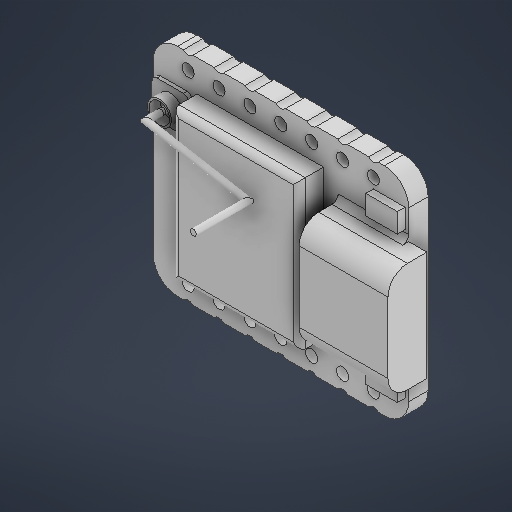
# Autodesk Inventor part: ESP32-S3
Saved by Autodesk Inventor 2027 (Build 310192000, 192)
## iProperties
Created: 2026-07-03
Part Number: ESP32-S3
Material: Genérico
Document SubType Name: Modeling
Designer: marcu
Density: 1 g/cm^3
Appearance: Padrão
Mass: 1.03876 g
Surface Area: 11.537 cm^2
Volume: 1.03876 cm^3
Author: marcu
Autodesk Inventor part; units mm, degrees
ref_plane "YZ Plane" through (0, 0, 0) normal (1, 0, 0) x (0, 1, 0)
ref_plane "XZ Plane" through (0, 0, 0) normal (0, 1, 0) x (-1, 0, 0)
sketch "Esboço1" plane through (0, 0, 0) normal (0, 0, 1) x (1, 0, 0)
  line L0 (-10.5, 8.9) -> (10.5, 8.9)
  line L1 (10.5, 8.9) -> (10.5, -8.9)
  line L2 (10.5, -8.9) -> (-10.5, -8.9)
  line L3 (-10.5, -8.9) -> (-10.5, 8.9)
  line L4 (-10.5, 8.9) -> (10.5, -8.9) construction
  line L5 (10.5, 8.9) -> (-10.5, -8.9) construction
  point P0 (0, 0)
  dimension "d0" = 21
  dimension "d1" = 17.8
  constraints: 12 end point, 2 midpoint, 2 parallel, 1 horizontal, 1 perpendicular
  measures "d0" distance of L1.end L2.end
  measures "d1" distance of L0.end L1.end
extrude "Extrusão1" add sketch "Esboço1" along normal mid plane 1.6
sketch "Esboço2" plane through (0, 0, 0.8) normal (0, 0, 1) x (1, 0, 0)
  line L0 (-23.9402, 0) -> (23.9402, 0) construction
  circle A0 centre (-7.63, 7.62) radius 0.5
  line L1 (-10.5, 8.9) -> (-10.5, -8.9) projected
  line L2 (10.5, 8.9) -> (-10.5, 8.9) projected
  circle A1 centre (-5.09, 7.62) radius 0.5
  circle A2 centre (-2.55, 7.62) radius 0.5
  circle A3 centre (-0.01, 7.62) radius 0.5
  circle A4 centre (2.53, 7.62) radius 0.5
  circle A5 centre (5.07, 7.62) radius 0.5
  circle A6 centre (7.61, 7.62) radius 0.5
  circle A7 centre (-7.63, -7.62) radius 0.5
  line L3 (10.5, -8.9) -> (-10.5, -8.9)
  circle A8 centre (-5.09, -7.62) radius 0.5
  circle A9 centre (-2.55, -7.62) radius 0.5
  circle A10 centre (-0.01, -7.62) radius 0.5
  circle A11 centre (2.53, -7.62) radius 0.5
  circle A12 centre (5.07, -7.62) radius 0.5
  circle A13 centre (7.61, -7.62) radius 0.5
  point P0 (0, 0)
  dimension "d4" = 1
  dimension "d13" = 2.87
  dimension "d14" = 1.28
  dimension "d17" = 2.54
  constraints: 14 centre point, 8 symmetric about line, 4 end point, 2 horizontal, 1 midpoint, 19 other
  measures "d4" diameter of A0
  measures "d13" distance from line of L1 A0.centre
  measures "d14" distance from line of L2 A0.centre
  measures "d17" distance of A0.centre A1.centre
extrude "Extrusão2" cut sketch "Esboço2" against normal blind 2
fillet "Arredondamento1" radius 2 2 edges at (-10.5, 8.9, 0) (-10.5, -8.9, 0)
fillet "Arredondamento2" radius 2 2 edges at (10.5, -8.9, 0) (10.5, 8.9, 0)
sketch "Esboço3" plane through (0, 0, 0.8) normal (0, 0, 1) x (1, 0, 0)
  line L0 (12, -11.9784) -> (12, 11.9784) construction
  line L1 (10.5, -6.9) -> (10.5, 6.9) projected
  line L2 (12, -4.5) -> (4.7, -4.5)
  line L3 (4.7, -4.5) -> (4.7, 4.5)
  line L4 (4.7, 4.5) -> (12, 4.5)
  line L5 (12, 4.5) -> (12, -4.5)
  line L6 (-8.5, -8.9) -> (8.5, -8.9) projected
  point P0 (0, 0)
  dimension "d26" = 1.5
  dimension "d27" = 9
  dimension "d28" = 7.3
  dimension "d29" = 4.4
  constraints: 10 end point, 2 parallel, 2 perpendicular, 1 point on line, 1 vertical
  measures "d26" distance between parallel lines of L1 L0
  measures "d27" distance of L2.end L3.end
  measures "d28" distance of L2.start L2.end
  measures "d29" distance between parallel lines of L2 L6
extrude "Extrusão3" add sketch "Esboço3" along normal blind 3.2
fillet "Arredondamento4" radius 1.6 2 edges at (8.35, 4.5, 4) (8.35, -4.5, 4)
fillet "Arredondamento5" radius 0.5 2 edges at (7.6, -4.5, 0.8) (7.6, 4.5, 0.8)
sketch "Esboço4" plane through (0, 0, 0.8) normal (0, 0, 1) x (1, 0, 0)
  line L0 (-8.5, -8.9) -> (8.5, -8.9) projected
  circle A0 centre (7.61, -9.22) radius 0.5
  line L1 (8.3896, -8.72) -> (6.8304, -8.72) construction
  circle A1 centre (7.61, -7.62) radius 0.5 projected
  line L2 (8.5997, -8.12) -> (6.6203, -8.12) construction
  line L3 (10.5, -6.9) -> (10.5, -5) projected
  circle A2 centre (5.07, -9.22) radius 0.5
  line L4 (5.8496, -8.72) -> (4.2904, -8.72) construction
  circle A3 centre (2.53, -9.22) radius 0.5
  line L5 (3.3096, -8.72) -> (1.7504, -8.72) construction
  circle A4 centre (-0.01, -9.22) radius 0.5
  line L6 (0.7696, -8.72) -> (-0.7896, -8.72) construction
  circle A5 centre (-2.55, -9.22) radius 0.5
  line L7 (-1.7704, -8.72) -> (-3.3296, -8.72) construction
  circle A6 centre (-5.09, -9.22) radius 0.5
  line L8 (-4.3104, -8.72) -> (-5.8696, -8.72) construction
  circle A7 centre (-7.63, -9.22) radius 0.5
  line L9 (-6.8504, -8.72) -> (-8.4096, -8.72) construction
  line L10 (2.05, 0) -> (-2.05, 0) construction
  line L11 (-8.5, 8.9) -> (8.5, 8.9)
  circle A8 centre (7.61, 9.22) radius 0.5
  line L12 (8.3896, 8.72) -> (6.8304, 8.72) construction
  circle A9 centre (5.07, 9.22) radius 0.5
  line L13 (5.8496, 8.72) -> (4.2904, 8.72) construction
  circle A10 centre (2.53, 9.22) radius 0.5
  line L14 (3.3096, 8.72) -> (1.7504, 8.72) construction
  circle A11 centre (-0.01, 9.22) radius 0.5
  line L15 (0.7696, 8.72) -> (-0.7896, 8.72) construction
  circle A12 centre (-2.55, 9.22) radius 0.5
  line L16 (-1.7704, 8.72) -> (-3.3296, 8.72) construction
  circle A13 centre (-5.09, 9.22) radius 0.5
  line L17 (-4.3104, 8.72) -> (-5.8696, 8.72) construction
  circle A14 centre (-7.63, 9.22) radius 0.5
  line L18 (-6.8504, 8.72) -> (-8.4096, 8.72) construction
  point P0 (0, 0)
  point P1 (7.61, -8.72)
  point P2 (7.61, -8.12)
  point P3 (5.96, -8.9)
  point P4 (5.07, -8.72)
  point P5 (3.42, -8.9)
  point P6 (2.53, -8.72)
  point P7 (0.88, -8.9)
  point P8 (-0.01, -8.72)
  point P9 (-1.66, -8.9)
  point P10 (-2.55, -8.72)
  point P11 (-4.2, -8.9)
  point P12 (-5.09, -8.72)
  point P13 (-6.74, -8.9)
  point P14 (-7.63, -8.72)
  point P15 (7.61, 8.72)
  point P16 (5.96, 8.9)
  point P17 (5.07, 8.72)
  point P18 (3.42, 8.9)
  point P19 (2.53, 8.72)
  point P20 (0.88, 8.9)
  point P21 (-0.01, 8.72)
  point P22 (-1.66, 8.9)
  point P23 (-2.55, 8.72)
  point P24 (-4.2, 8.9)
  point P25 (-5.09, 8.72)
  point P26 (-6.74, 8.9)
  point P27 (-7.63, 8.72)
  dimension "d36" = 1
  dimension "d37" = 0.6
  dimension "d38" = 2.39
  dimension "d41" = 2.54
  constraints: 36 symmetric about line, 34 end point, 19 horizontal, 15 vertical alignment, 3 midpoint, 65 other
  measures "d37" distance between parallel lines of L2 L1
  measures "d41" distance of L0.end point (5.96, -8.9)
extrude "Extrusão4" cut sketch "Esboço4" against normal blind 3.2 contours A7 L0 | L0 A7 | A6 L0 | L0 A6 | A5 L0 | L0 A5 | A4 L0 | L0 A4 | A3 L0 | L0 A3 | A2 L0 | L0 A2 | A0 L0 | L0 A0 | A14 L11 | L11 A14 | A13 L11 | L11 A13 | A12 L11 | L11 A12 | A11 L11 | L11 A11 | A10 L11 | L11 A10 | A9 L11 | L11 A9 | A8 L11 | L11 A8
sketch "Esboço5" plane through (0, 0, 0.8) normal (0, 0, 1) x (1, 0, 0)
  line L0 (3.5, -5.9) -> (3.5, 6.7)
  line L1 (4.7, -5) -> (4.7, 5) projected
  line L2 (3.5, -5.9) -> (-6.9, -5.9)
  line L3 (-6.9, -5.9) -> (-6.9, 6.3)
  line L4 (-6.9, 6.3) -> (3.5, 6.3)
  line L5 (3.5, 6.3) -> (3.5, -5.9)
  line L6 (-0.3942, 8.9) -> (-2.1658, 8.9) projected
  point P0 (0, 0)
  point P1 (-1.28, 8.9)
  point P2 (3.5, 6.3)
  dimension "d52" = 1.2
  dimension "d53" = 10.4
  dimension "d56" = 12.2
  dimension "d57" = 2.6
  constraints: 10 end point, 2 parallel, 1 horizontal, 1 midpoint, 1 perpendicular, 1 vertical
  measures "d52" distance between parallel lines of L0 L1
  measures "d53" distance of L0.start L2.end
  measures "d56" distance between parallel lines of L4 L2
  measures "d57" distance from line of point (-1.28, 8.9) L4
extrude "Extrusão5" add sketch "Esboço5" along normal blind 2
fillet "Arredondamento6" radius 0.5 4 edges at (-1.7, -5.9, 2.8) (-1.7, 6.3, 2.8) (3.5, 0.2, 2.8) (-6.9, 0.2, 2.8)
sketch "Esboço6" plane through (0, 0, 0.8) normal (0, 0, 1) x (1, 0, 0)
  line L0 (-7.3, 6.1) -> (-10.3, 6.1)
  line L1 (-10.3, 6.1) -> (-10.3, 3.1)
  line L2 (-10.3, 3.1) -> (-7.3, 3.1)
  line L3 (-7.3, 3.1) -> (-7.3, 6.1)
  line L4 (-7.3, 6.1) -> (-10.3, 3.1) construction
  line L5 (-10.3, 6.1) -> (-7.3, 3.1) construction
  line L6 (-8.0142, 8.9) -> (-8.5, 8.9) projected
  line L7 (-6.9, -5.9) -> (-6.9, 6.3) projected
  point P0 (0, 0)
  point P1 (-8.8, 4.6)
  point P2 (-8.2571, 8.9)
  dimension "d61" = 3
  dimension "d62" = 3
  dimension "d63" = 2.8
  dimension "d64" = 0.4
  constraints: 12 end point, 3 midpoint, 2 parallel, 1 horizontal, 1 perpendicular
  measures "d61" distance of L2.end L1.end
  measures "d62" distance of L1.end L0.end
  measures "d63" distance from line of point (-8.257, 8.9) L0
  measures "d64" distance between parallel lines of L3 L7
extrude "Extrusão6" add sketch "Esboço6" along normal blind 0.3
fillet "Arredondamento7" radius 0.4 4 edges at (-10.3, 3.1, 0.95) (-7.3, 3.1, 0.95) (-10.3, 6.1, 0.95) (-7.3, 6.1, 0.95)
sketch "Esboço7" plane through (0, 0, 1.1) normal (0, 0, 1) x (1, 0, 0)
  circle A0 centre (-8.8, 4.6) radius 1
  line L0 (-7.3, 3.5) -> (-7.3, 5.7) projected
  line L1 (-7.7, 6.1) -> (-9.9, 6.1) projected
  point P0 (0, 0)
  point P1 (-8.8, 6.1)
  dimension "d68" = 2
  dimension "d69" = 0.5
  dimension "d70" = 1.5
  constraints: 1 centre point, 1 midpoint
  measures "d68" diameter of A0
  measures "d69" distance edge to line of A0 L0
  measures "d70" distance of point (-8.8, 6.1) A0.centre
extrude "Extrusão7" add sketch "Esboço7" along normal blind 0.9
sketch "Esboço8" plane through (-8.8, 4.6, 2) normal (0, 0, 1) x (1, 0, 0)
  circle A0 centre (0, 0) radius 0.85
  circle A1 centre (0, 0) radius 1 projected
  point P0 (8.8, -4.6)
  dimension "d73" = 1.7
  dimension "d75" = 0.15
  constraints: 1 centre point
  measures "d73" diameter of A0
  measures "d75" radial gap between concentric circles of A1 A0
extrude "Extrusão8" cut sketch "Esboço8" against normal blind 0.9 contours A0
sketch "Esboço9" plane through (-8.8, 4.6, 1.1) normal (0, 0, 1) x (1, 0, 0)
  circle A0 centre (0, 0) radius 0.85 projected
  circle A1 centre (0, 0) radius 0.25
  point P0 (8.8, -4.6)
  dimension "d82" = 0.5
  constraints: 1 centre point, 1 coincident
  measures "d82" diameter of A1
extrude "Extrusão10" add sketch "Esboço9" along normal blind 0.8 contours A1
fillet "Arredondamento8" radius 0.2 1 edges at (-9.05, 4.6, 1.9)
sketch "Esboço10" plane through (0, 0, 0.8) normal (0, 0, 1) x (1, 0, 0)
  line L0 (10.2, -5.2) -> (7.6, -5.2)
  line L1 (7.6, -5.2) -> (7.6, -6.8)
  line L2 (7.6, -6.8) -> (10.2, -6.8)
  line L3 (10.2, -6.8) -> (10.2, -5.2)
  line L4 (10.2, -5.2) -> (7.6, -6.8) construction
  line L5 (7.6, -5.2) -> (10.2, -6.8) construction
  line L6 (7.9942, -8.9) -> (8.5, -8.9) projected
  line L7 (10.5, -6.9) -> (10.5, -5) projected
  line L8 (16.9434, 0) -> (12.9434, 0) construction
  line L9 (10.2, 5.2) -> (7.6, 5.2)
  line L10 (7.6, 5.2) -> (7.6, 6.8)
  line L11 (7.6, 6.8) -> (10.2, 6.8)
  line L12 (10.2, 6.8) -> (10.2, 5.2)
  line L13 (10.2, 5.2) -> (7.6, 6.8) construction
  line L14 (7.6, 5.2) -> (10.2, 6.8) construction
  line L15 (10.5, 6.9) -> (10.5, 5)
  point P0 (0, 0)
  point P1 (8.9, -6)
  point P2 (8.2471, -8.9)
  point P3 (8.9, 6)
  dimension "d86" = 2.6
  dimension "d87" = 1.6
  dimension "d88" = 2.1
  dimension "d89" = 0.3
  dimension "d90" = 4
  dimension "d91" = 8.9
  dimension "d92" = 6.4434
  constraints: 28 end point, 7 symmetric about line, 3 midpoint, 2 horizontal, 2 parallel, 1 perpendicular
  measures "d86" distance of L2.end L1.end
  measures "d87" distance of L1.end L0.end
  measures "d88" distance from line of point (8.247, -8.9) L2
  measures "d89" distance between parallel lines of L3 L7
  measures "d90" distance of L8.start L8.end
  measures "d91" distance between parallel lines of L8 L6
  measures "d92" distance from line of L8.start L7
extrude "Extrusão11" add sketch "Esboço10" along normal blind 0.63
ref_plane "Plano de trabalho1" through (0, 0, 8) normal (0, 0, 1) x (1, 0, 0)
sketch "Esboço12" plane through (0, 0, 8) normal (0, 0, 1) x (1, 0, 0)
  line L0 (0, 0) -> (0, 3.5) construction
  circle A0 centre (0, 3.5) radius 0.25
  dimension "d97" = 3.5
  dimension "d98" = 0.5
  constraints: 2 end point, 1 centre point, 1 coincident, 1 vertical
  measures "d97" distance of L0.start L0.end
  measures "d98" diameter of A0
sketch3d "Esboço 3D1"
  line L0 (0, 3.5, 8) -> (0, 3.5, 3.5)
  line L1 (0, 3.5, 3.5) -> (-8.8, 4.6, 3.1)
  line L2 (-8.8, 4.6, 3.1) -> (-8.8, 4.6, 1.9)
  dimension "d99" = 1.2
  dimension "d100" = 4.5
sweep "Antena" add profiles "Esboço12" path "Esboço 3D1"
